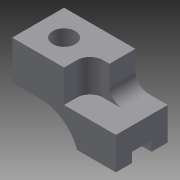
# Autodesk Inventor part: HW 8 Part 1
Saved by Autodesk Inventor 2015 (Build 190159000, 159)
## iProperties
Created: 2016-03-08
Part Number: HW 8 Part 1
Material: Generic
Document SubType Name: Modeling
Designer: Melissa
Density: 1 g/cm^3
Appearance: Default
Author: Melissa
Autodesk Inventor part; units mm, degrees
ref_plane "YZ Plane" through (0, 0, 0) normal (1, 0, 0) x (0, 1, 0)
ref_plane "XZ Plane" through (0, 0, 0) normal (0, 1, 0) x (-1, 0, 0)
ref_plane "XY Plane" through (0, 0, 0) normal (0, 0, 1) x (1, 0, 0)
sketch "Sketch1" plane through (0, 0, 0) normal (0, 0, 1) x (1, 0, 0)
  line L0 (0, 0) -> (0, 76.2)
  line L1 (0, 76.2) -> (139.7, 76.2)
  line L2 (139.7, 76.2) -> (139.7, 38.1)
  line L3 (165.1, 12.7) -> (203.2, 12.7)
  line L4 (203.2, 12.7) -> (203.2, -50.8)
  line L5 (203.2, -50.8) -> (127, -50.8)
  line L6 (0, 0) -> (55.158, 0)
  arc A0 (139.7, 38.1) -> (165.1, 12.7) centre (165.1, 38.1) ccw
  arc A1 (127, -50.8) -> (55.158, 0) centre (55.158, -76.2) ccw
  dimension "d0" = 76.2
  dimension "d2" = 203.2
  dimension "d3" = 139.7
  dimension "d4" = 76.2
  dimension "d5" = 127
  dimension "d6" = 63.5
  dimension "d7" = 25.4
  dimension "d8" = 76.2
  constraints: 14 end point, 5 perpendicular, 4 point on circle, 3 tangent, 2 centre point, 1 horizontal, 1 vertical
  measures "d0" distance of L0.start L0.end
  measures "d2" horizontal distance of L3.end L0.end
  measures "d3" distance of L0.end L1.end
  measures "d4" distance of L4.end L5.end
  measures "d5" horizontal distance of L5.end L0.end
  measures "d6" distance of L3.end L4.end
  measures "d7" radius of A0
  measures "d8" radius of A1
extrude "Extrusion1" add sketch "Sketch1" along normal blind 101.6
sketch "Sketch2" plane through (0, 76.2, 0) normal (0, 1, 0) x (1, 0, 0)
  line L0 (139.7, 0) -> (139.7, -50.8)
  line L1 (139.7, 0) -> (139.7, -101.6) projected
  line L2 (0, -101.6) -> (101.6, -101.6)
  line L3 (127, -101.6) -> (55.158, -101.6) projected
  line L4 (101.6, -101.6) -> (101.6, -76.2)
  line L5 (127, -50.8) -> (139.7, -50.8)
  arc A0 (127, -50.8) -> (101.6, -76.2) centre (127, -76.2) ccw
  line L6 (101.6, -101.6) -> (139.7, -101.6)
  line L7 (139.7, -101.6) -> (165.1, -101.6)
  line L8 (165.1, -101.6) -> (165.1, -50.8)
  line L9 (165.1, 0) -> (165.1, -101.6) projected
  line L10 (165.1, -50.8) -> (139.7, -50.8)
  point P0 (0, 0)
  dimension "d11" = 50.8
  dimension "d12" = 101.6
  dimension "d13" = 25.4
  constraints: 16 end point, 3 horizontal, 2 midpoint, 2 point on circle, 2 tangent, 1 centre point, 1 collinear, 1 perpendicular, 1 point on line
  measures "d11" distance of L0.start L0.end
  measures "d12" distance of L2.start L2.end
  measures "d13" radius of A0
extrude "Extrusion3" cut sketch "Sketch2" against normal blind 63.5
sketch "Sketch3" plane through (0, 76.2, 0) normal (0, 1, 0) x (1, 0, 0)
  circle A0 centre (50.8, -50.8) radius 22.225
  line L0 (55.158, 0) -> (0, 0) projected
  line L1 (0, 0) -> (0, -101.6) projected
  dimension "d18" = 44.45
  dimension "d19" = 50.8
  dimension "d20" = 50.8
  constraints: 1 centre point
  measures "d18" diameter of A0
  measures "d19" distance from line of L0 A0.centre
  measures "d20" distance from line of A0.centre L1
extrude "Extrusion4" cut sketch "Sketch3" against normal through all
sketch "Sketch4" plane through (203.2, -50.8, 0) normal (1, 0, 0) x (0, 0, -1)
  line L0 (0, 0) -> (-31.75, 0)
  line L1 (0, 0) -> (-101.6, 0) projected
  line L2 (-31.75, 0) -> (-31.75, 19.05)
  line L3 (-31.75, 19.05) -> (-69.85, 19.05)
  line L4 (-69.85, 19.05) -> (-69.85, 0)
  line L5 (-31.75, 0) -> (-69.85, 0)
  point P0 (0, 50.8)
  dimension "d23" = 31.75
  dimension "d24" = 19.05
  dimension "d25" = 38.1
  constraints: 10 end point, 2 perpendicular, 2 point on line, 1 collinear, 1 vertical
  measures "d23" distance of L0.start L0.end
  measures "d24" distance of L0.end L2.end
  measures "d25" distance of L2.end L3.end
extrude "Extrusion5" cut sketch "Sketch4" against normal through all
body "Solid1"
